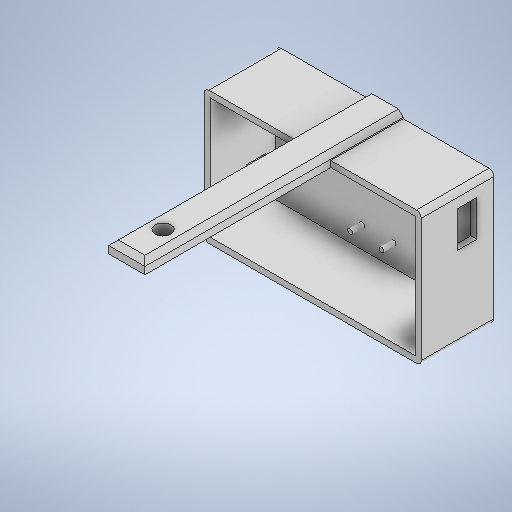
# Autodesk Inventor part: adapter_box
Saved by Autodesk Inventor 2025 (Build 290162000, 162)
## iProperties
Created: 2025-02-26
Part Number: adapter_box
Material: Všeobecné
Document SubType Name: Modeling
Designer: lukas
Density: 1 g/cm^3
Appearance: Výchozí
Author: lukas
## iProperties of the stored document adapter_box_3D tisk.ipt
Created: 2025-02-26
Part Number: adapter_box_3D tisk
Material: Všeobecné
Document SubType Name: Modeling
Designer: lukas
Density: 1 g/cm^3
Appearance: Výchozí
Author: lukas
Autodesk Inventor part; units mm, degrees
ref_plane "YZ Plane" through (0, 0, 0) normal (1, 0, 0) x (0, 1, 0)
ref_plane "XZ Plane" through (0, 0, 0) normal (0, 1, 0) x (-1, 0, 0)
ref_plane "XY Plane" through (0, 0, 0) normal (0, 0, 1) x (1, 0, 0)
sketch "Náčrt1" plane through (0, 0, 0) normal (0, 0, 1) x (1, 0, 0)
  line L0 (0, 35) -> (0, -35) projected
  line L1 (-59.5, 0) -> (59.5, 0) projected
  line L2 (42.5, -25) -> (-42.5, -25)
  line L3 (-42.5, -25) -> (-42.5, 25)
  line L4 (-42.5, 25) -> (42.5, 25)
  line L5 (42.5, 25) -> (42.5, -25)
  point P0 (0, 0)
  dimension "d1" = 85
  dimension "d2" = 50
  constraints: 8 end point, 2 parallel, 1 horizontal, 1 perpendicular, 2 other
  measures "d1" distance of L3.end L4.end
  measures "d2" distance between parallel lines of L2 L4
extrude "Vysunutí1" add sketch "Náčrt1" along normal blind 3
sketch "Náčrt2" plane through (0, 0, 0) normal (0, 0, -1) x (-1, 0, 0)
  line L0 (-42.5, 25) -> (42.5, 25) projected
  line L1 (-42.5, -25) -> (-42.5, 25) projected
  line L2 (42.5, -25) -> (-42.5, -25) projected
  line L3 (42.5, 25) -> (42.5, -25) projected
  line L4 (45, 27.5) -> (-45, 27.5)
  line L5 (-45, 27.5) -> (-45, -27.5)
  line L6 (-45, -27.5) -> (45, -27.5)
  line L7 (45, -27.5) -> (45, 27.5)
  line L8 (-42.5, 25) -> (42.5, 25)
  line L9 (42.5, 25) -> (42.5, -25)
  line L10 (42.5, -25) -> (-42.5, -25)
  line L11 (-42.5, -25) -> (-42.5, 25)
  point P0 (0, 0)
  dimension "d5" = 2.5
  constraints: 16 end point, 2 parallel, 1 horizontal, 1 perpendicular, 3 other
  measures "d5" distance between parallel lines of L0 L4
extrude "Vysunutí2" add sketch "Náčrt2" against normal blind 30
sketch "Náčrt3" plane through (0, 0, 3) normal (0, 0, 1) x (1, 0, 0)
  line L0 (42.5, 25) -> (-42.5, 25) projected
  line L1 (-42.5, 25) -> (-42.5, -25) projected
  line L2 (-42.5, -25) -> (42.5, -25) projected
  line L3 (42.5, -25) -> (42.5, 25) projected
  line L4 (0, 35) -> (0, -35) projected
  line L5 (-63, 0) -> (63, 0) projected
  line L6 (2.5, 21.5) -> (37.5, 21.5) construction
  line L7 (37.5, 21.5) -> (37.5, -21.5) construction
  line L8 (37.5, -21.5) -> (2.5, -21.5) construction
  line L9 (2.5, -21.5) -> (2.5, 21.5) construction
  line L10 (-2.5, 21.5) -> (-37.5, 21.5) construction
  line L11 (-37.5, 21.5) -> (-37.5, -21.5) construction
  line L12 (-37.5, -21.5) -> (-2.5, -21.5) construction
  line L13 (-2.5, -21.5) -> (-2.5, 21.5) construction
  circle A0 centre (6.5, 16) radius 1
  circle A1 centre (6.5, -16) radius 1
  circle A2 centre (-6.5, 16) radius 1
  circle A3 centre (-6.5, -16) radius 1
  point P0 (0, 0)
  point P1 (9, -16)
  dimension "d8" = 35
  dimension "d9" = 43
  dimension "d10" = 3.5
  dimension "d11" = 5
  dimension "d15" = 2
  dimension "d16" = 36
  dimension "d17" = 16
  constraints: 16 end point, 7 symmetric about line, 4 centre point, 2 parallel, 1 horizontal, 1 perpendicular, 3 other
  measures "d8" distance of L6.start L6.end
  measures "d9" distance of L6.end L7.end
  measures "d10" distance between parallel lines of L0 L6
  measures "d11" distance between parallel lines of L3 L7
  measures "d15" diameter of A0
  measures "d16" distance from line of L3 A0.centre
  measures "d17" distance from line of L5 A0.centre
extrude "Vysunutí3" add sketch "Náčrt3" along normal blind 5 contours A0 | A1 | A2 | A3
sketch "Náčrt4" plane through (45, -27.5, 0) normal (1, 0, 0) x (0, 0, -1)
  line L0 (-3, 2.5) -> (-3, 52.5) projected
  line L1 (0, 55) -> (0, 0) projected
  line L2 (0, 55) -> (-30, 55) projected
  line L3 (-30, 0) -> (-30, 55) projected
  line L4 (0, 0) -> (-30, 0) projected
  line L5 (-36, 27.5) -> (6, 27.5) projected
  line L6 (0, -11) -> (0, 66) projected
  line L7 (-7, 34) -> (-15, 34)
  line L8 (-15, 34) -> (-15, 49)
  line L9 (-15, 49) -> (-7, 49)
  line L10 (-7, 49) -> (-7, 34)
  point P0 (0, 27.5)
  point P1 (-3, 34)
  point P2 (-3, 49)
  dimension "d20" = 8
  dimension "d21" = 15
  dimension "d22" = 6
  dimension "d24" = 7
  constraints: 8 end point, 2 parallel, 1 horizontal, 1 perpendicular
  measures "d20" distance of L8.end L9.end
  measures "d21" distance of L7.end L8.end
  measures "d22" distance between parallel lines of L9 L2
  measures "d24" distance between parallel lines of L1 L10
extrude "Vysunutí4" cut sketch "Náčrt4" against normal up to surface (2.5 mm away) contours L7 L8 L9 L10
pattern_circular "Kruhové pole1" count 2 over 360 about axis through (0, 0, -10) along (0, 0, 1) of "Vysunutí4"
sketch "Náčrt5" plane through (-45, 27.5, 0) normal (0, 1, 0) x (1, 0, 0)
  line L0 (0, 0) -> (90, 0) projected
  line L1 (0, 0) -> (0, -30) projected
  line L2 (90, -30) -> (0, -30) projected
  line L3 (90, 0) -> (90, -30) projected
  line L4 (-18, 0) -> (108, 0) projected
  line L5 (45, 6) -> (45, -36) projected
  line L6 (37.5, -30) -> (52.5, -30)
  line L7 (52.5, -30) -> (52.5, -107)
  line L8 (52.5, -107) -> (37.5, -107)
  line L9 (37.5, -107) -> (37.5, -30)
  line L10 (0, 0) -> (90, 0) projected
  line L11 (52.5, -30) -> (37.5, -30)
  line L12 (37.5, -30) -> (37.5, 0)
  line L13 (37.5, 0) -> (52.5, 0)
  line L14 (52.5, 0) -> (52.5, -30)
  point P0 (45, 0)
  dimension "d31" = 77
  dimension "d32" = 15
  dimension "d33" = 15
  constraints: 16 end point, 4 parallel, 2 horizontal, 2 perpendicular, 2 point on line, 1 other
  measures "d31" distance of L8.end L6.start
  measures "d32" distance of L7.end L8.end
  measures "d33" distance between parallel lines of L14 L12
extrude "Vysunutí5" add sketch "Náčrt5" along normal mid plane 5 contours L0 L5 L2 L12 | L0 L14 L2 L5 | L2 L7 L8 L9
fillet "Zaoblení1" radius 2 4 edges at (-45, 27.5, 15) (-45, -27.5, 15) (45, -27.5, 15) (45, 27.5, 15)
sketch "Náčrt6" plane through (-45, 30, 0) normal (0, 1, 0) x (1, 0, 0)
  line L0 (37.5, -107) -> (52.5, -107) projected
  line L1 (52.5, -107) -> (52.5, 0) projected
  line L2 (52.5, 0) -> (37.5, 0) projected
  line L3 (37.5, 0) -> (37.5, -107) projected
  point P0 (45, 0)
  point P1 (45, -92)
  point P2 (45, -107)
  dimension "d37" = 7.5
  dimension "d38" = 15
  constraints: 1 midpoint
  measures "d37" distance from line of L3 point (45, -92)
  measures "d38" distance of point (45, -107) point (45, -92)
hole "Díra1" at (0, 30, 92) direction (0, -1, 0) diameter 6.6 end through all
chamfer "Zkosení1" distance 2 angle 45 3 edges at (7.5, 30, 53.5) (-7.5, 30, 53.5) (0, 30, 107)
